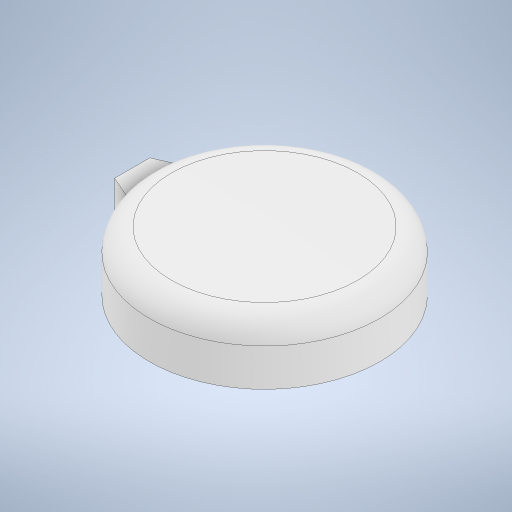
# Autodesk Inventor part: GPSR_antenna
Saved by Autodesk Inventor 2023 (Build 270158000, 158)
## iProperties
Created: 2023-06-07
Part Number: GPSR_antenna
Material: ABS Plastic
Document SubType Name: Modeling
Designer: 310611102
Density: 3.18261 g/cm^3
Appearance: Smooth - White
Mass: 92.18 g
Surface Area: 57.3858 cm^2
Volume: 28.9636 cm^3
Author: 310611102
Autodesk Inventor part; units mm, degrees
ref_plane "YZ Plane" through (0, 0, 0) normal (1, 0, 0) x (0, 1, 0)
ref_plane "XZ Plane" through (0, 0, 0) normal (0, 1, 0) x (-1, 0, 0)
ref_plane "XY Plane" through (0, 0, 0) normal (0, 0, 1) x (1, 0, 0)
sketch "Sketch1" plane through (0, 0, 0) normal (0, 0, 1) x (1, 0, 0)
  line L0 (0, 0) -> (0, 13.5)
  line L1 (0, 13.5) -> (21.1, 13.5)
  line L2 (26.1, 8.5) -> (26.1, 0)
  line L3 (26.1, 0) -> (0, 0)
  line L4 (0, 0) -> (0, 45.7407)
  arc A0 (26.1, 8.5) -> (21.1, 13.5) centre (21.1, 8.5) ccw
  dimension "d2" = 52.2
  dimension "d3" = 13.5
  dimension "d4" = 5
  constraints: 10 end point, 3 perpendicular, 2 point on circle, 2 tangent, 2 vertical, 1 centre point
  measures "d2" diameter of L2 L4
  measures "d3" distance between parallel lines of L3 L1
  measures "d4" radius of A0
revolve "Revolution1" add sketch "Sketch1" angle 360 about axis through (0, 0, 0) along (0, 1, 0)
sketch "Sketch2" plane through (0, 0, 0) normal (0, -1, 0) x (1, 0, 0)
  circle A0 centre (0, 0) radius 26.1 projected
  line L0 (-25.401, -6) -> (-30, -4)
  line L1 (-30, -4) -> (-30, 4)
  line L2 (-30, 4) -> (-25.401, 6)
  line L3 (-25.401, 6) -> (-25.401, -6)
  point P0 (-30, 0)
  dimension "d6" = 8
  dimension "d7" = 12
  dimension "d8" = 30
  constraints: 8 end point, 2 point on circle, 2 vertical, 1 horizontal alignment, 1 midpoint
  measures "d6" distance of L0.end L1.end
  measures "d7" distance of L2.end L0.start
  measures "d8" distance from line of point (0, 0) L1
extrude "Extrusion1" add sketch "Sketch2" against normal blind 10 contours A0 L0 L1 L2
sketch "Sketch3" plane through (-30, 0, -4) normal (-1, 0, 0) x (0, 0, 1)
  circle A0 centre (4, 7) radius 1.35
  line L0 (8, 0) -> (0, 0) projected
  point P0 (4, 0)
  point P1 (4, 0)
  point P2 (4, 0)
  dimension "d11" = 2.7
  dimension "d12" = 7
  constraints: 2 midpoint, 1 centre point, 1 vertical alignment
  measures "d11" diameter of A0
  measures "d12" distance of point (4, 0) A0.centre
body "Solid1"
